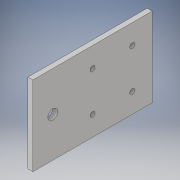
# Autodesk Inventor part: 2AM-17-P-0206  - slider plate
Saved by Autodesk Inventor 2017 (Build 210142000, 142)
## iProperties
Created: 2017-12-27
Part Number: 2AM-17-P-0206  - slider plate
Material: Generic
Document SubType Name: Modeling
Designer: Micah
Density: 1 g/cm^3
Appearance: Default
Author: Micah
Autodesk Inventor part; units mm, degrees
ref_plane "YZ Plane" through (0, 0, 0) normal (1, 0, 0) x (0, 1, 0)
ref_plane "XZ Plane" through (0, 0, 0) normal (0, 1, 0) x (-1, 0, 0)
ref_plane "XY Plane" through (0, 0, 0) normal (0, 0, 1) x (1, 0, 0)
sketch "Sketch1" plane through (0, 0, 0) normal (1, 0, 0) x (0, 1, 0)
  line L0 (0, 0) -> (50.8, 0)
  line L1 (50.8, 0) -> (50.8, 76.2)
  line L2 (50.8, 76.2) -> (0, 76.2)
  line L3 (0, 76.2) -> (0, 0)
  line L4 (50.8, 0) -> (50.8, 50.8) construction
  line L5 (50.8, 50.8) -> (0, 50.8) construction
  line L6 (50.8, 0) -> (50.8, 12.7) construction
  line L7 (50.8, 12.7) -> (38.1, 12.7) construction
  line L8 (0, 12.7) -> (12.7, 12.7) construction
  circle A0 centre (12.7, 12.7) radius 1.5875
  circle A1 centre (38.1, 12.7) radius 1.5875
  line L9 (50.8, 12.7) -> (50.8, 38.1) construction
  line L10 (50.8, 25.4) -> (0, 25.4) construction
  circle A2 centre (12.7, 38.1) radius 1.5875
  circle A3 centre (38.1, 38.1) radius 1.5875
  line L11 (50.8, 76.2) -> (50.8, 63.5) construction
  line L12 (50.8, 63.5) -> (0, 63.5) construction
  line L13 (25.4, 76.2) -> (25.4, 63.5) construction
  circle A4 centre (25.4, 63.5) radius 3.175
  dimension "d0" = 50.8
  dimension "d1" = 76.2
  dimension "d2" = 50.8
  dimension "d3" = 12.7
  dimension "d4" = 12.7
  dimension "d5" = 12.7
  dimension "d6" = 3.175
  dimension "d7" = 3.175
  dimension "d8" = 12.7
  dimension "d9" = 6.35
  constraints: 28 end point, 8 point on line, 6 perpendicular, 5 centre point, 3 coincident, 3 midpoint, 2 parallel, 2 symmetric about line, 1 horizontal, 2 other
  measures "d0" distance of L2.end L1.end
  measures "d1" distance of L1.end L0.end
  measures "d2" distance of L0.end L4.end
  measures "d3" distance of L0.end L6.end
  measures "d4" distance of L6.end L7.end
  measures "d5" distance of L8.start L8.end
  measures "d6" diameter of A0
  measures "d7" diameter of A1
  measures "d8" distance of L1.end L11.end
  measures "d9" diameter of A4
extrude "Extrusion1" add sketch "Sketch1" along normal blind 3.175
body "Solid1"
